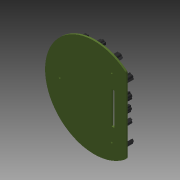
# Autodesk Inventor part: PCB
Saved by Autodesk Inventor 2015 (Build 190159000, 159)
## iProperties
Created: 2016-09-07
Part Number: PCB
Material: Generic
Document SubType Name: Modeling
Designer: James Yelland
Density: 1 g/cm^3
Appearance: Default
Author: James Yelland
Autodesk Inventor part; units mm, degrees
ref_plane "YZ Plane" through (0, 0, 0) normal (1, 0, 0) x (0, 1, 0)
ref_plane "XZ Plane" through (0, 0, 0) normal (0, 1, 0) x (-1, 0, 0)
ref_plane "XY Plane" through (0, 0, 0) normal (0, 0, 1) x (1, 0, 0)
sketch "Sketch4" plane through (0, 0, 0) normal (0, 1, 0) x (-1, 0, 0)
  line L0 (-55, 0) -> (-55, 62.45)
  line L1 (-55, 0) -> (-55, -62.45)
  arc A0 (-53.125, -66.3531) -> (-53.125, 66.3531) centre (0, 0) ccw
  arc A1 (-53.125, 66.3531) -> (-55, 62.45) centre (-50, 62.45) ccw
  arc A2 (-55, -62.45) -> (-53.125, -66.3531) centre (-50, -62.45) ccw
  circle A3 centre (-30.0153, 51.9527) radius 1.6
  circle A4 centre (60, 0) radius 1.6
  circle A5 centre (-30.0153, -51.9527) radius 1.6
  point P0 (-55, -64.8074)
  dimension "d56" = 3.2
  dimension "d57" = 3.2
  dimension "d58" = 3.2
  constraints: 7 point on circle, 6 centre point, 4 end point, 2 point on line
  measures "d56" diameter of A3
  measures "d57" diameter of A4
  measures "d58" diameter of A5
extrude "Extrusion2" add sketch "Sketch4" along normal blind 3
sketch "Sketch5" plane through (0, 3, 0) normal (0, 1, 0) x (1, 0, 0)
  line L0 (-78, 5) -> (-74, 5)
  line L1 (-74, 5) -> (-74, -5)
  line L2 (-74, -5) -> (-78, -5)
  arc A0 (-78, 2.5807) -> (-78, -2.5807) centre (-77.05, 0) ccw
  line L3 (-78, -5) -> (-78, -2.5807)
  line L4 (-78, 2.5807) -> (-78, 5)
  line L5 (-77.05, 0) -> (-85, 0)
  line L6 (-73.976, -25.2299) -> (-70.2805, -23.6992)
  line L7 (-70.2805, -23.6992) -> (-66.4537, -32.938)
  line L8 (-73.0502, -27.4651) -> (-73.976, -25.2299)
  line L9 (-66.4537, -32.938) -> (-70.1492, -34.4687)
  arc A1 (-73.0502, -27.4651) -> (-71.075, -32.2336) centre (-71.1849, -29.4858) ccw
  line L10 (-71.1849, -29.4858) -> (-78.5298, -32.5281)
  line L11 (-70.1492, -34.4687) -> (-71.075, -32.2336)
  line L12 (-58.6899, -51.6188) -> (-55.8614, -48.7904)
  line L13 (-55.8614, -48.7904) -> (-48.7904, -55.8614)
  line L14 (-56.9792, -53.3295) -> (-58.6899, -51.6188)
  line L15 (-48.7904, -55.8614) -> (-51.6188, -58.6899)
  arc A2 (-56.9792, -53.3295) -> (-53.3295, -56.9792) centre (-54.4826, -54.4826) ccw
  line L16 (-54.4826, -54.4826) -> (-60.1041, -60.1041)
  line L17 (-51.6188, -58.6899) -> (-53.3295, -56.9792)
  line L18 (-34.4687, -70.1492) -> (-32.938, -66.4537)
  line L19 (-32.938, -66.4537) -> (-23.6992, -70.2805)
  line L20 (-32.2336, -71.075) -> (-34.4687, -70.1492)
  line L21 (-23.6992, -70.2805) -> (-25.2299, -73.976)
  arc A3 (-32.2336, -71.075) -> (-27.4651, -73.0502) centre (-29.4858, -71.1849) ccw
  line L22 (-29.4858, -71.1849) -> (-32.5281, -78.5298)
  line L23 (-25.2299, -73.976) -> (-27.4651, -73.0502)
  line L24 (-5, -78) -> (-5, -74)
  line L25 (-5, -74) -> (5, -74)
  line L26 (-2.5807, -78) -> (-5, -78)
  line L27 (5, -74) -> (5, -78)
  arc A4 (-2.5807, -78) -> (2.5807, -78) centre (0, -77.05) ccw
  line L28 (0, -77.05) -> (0, -85)
  line L29 (5, -78) -> (2.5807, -78)
  line L30 (25.2299, -73.976) -> (23.6992, -70.2805)
  line L31 (23.6992, -70.2805) -> (32.938, -66.4537)
  line L32 (27.4651, -73.0502) -> (25.2299, -73.976)
  line L33 (32.938, -66.4537) -> (34.4687, -70.1492)
  arc A5 (27.4651, -73.0502) -> (32.2336, -71.075) centre (29.4858, -71.1849) ccw
  line L34 (29.4858, -71.1849) -> (32.5281, -78.5298)
  line L35 (34.4687, -70.1492) -> (32.2336, -71.075)
  line L36 (46.5147, -53.5858) -> (43.6863, -50.7574)
  line L37 (43.6863, -50.7574) -> (50.7574, -43.6863)
  line L38 (48.2254, -51.8751) -> (46.5147, -53.5858)
  line L39 (50.7574, -43.6863) -> (53.5858, -46.5147)
  arc A6 (48.2254, -51.8751) -> (51.8751, -48.2254) centre (49.3785, -49.3785) ccw
  line L40 (49.3785, -49.3785) -> (55, -55)
  line L41 (53.5858, -46.5147) -> (51.8751, -48.2254)
  line L42 (46.6194, -24.7224) -> (42.9239, -23.1916)
  line L43 (42.9239, -23.1916) -> (46.7507, -13.9528)
  line L44 (47.5453, -22.4872) -> (46.6194, -24.7224)
  line L45 (46.7507, -13.9528) -> (50.4463, -15.4836)
  arc A7 (47.5453, -22.4872) -> (49.5204, -17.7187) centre (47.6552, -19.7394) ccw
  line L46 (47.6552, -19.7394) -> (55, -22.7817)
  line L47 (50.4463, -15.4836) -> (49.5204, -17.7187)
  line L48 (48, -5) -> (44, -5)
  line L49 (44, -5) -> (44, 5)
  line L50 (48, -2.5807) -> (48, -5)
  line L51 (44, 5) -> (48, 5)
  arc A8 (48, -2.5807) -> (48, 2.5807) centre (47.05, 0) ccw
  line L52 (47.05, 0) -> (55, 0)
  line L53 (48, 5) -> (48, 2.5807)
  line L54 (50.4463, 15.4836) -> (46.7507, 13.9528)
  line L55 (46.7507, 13.9528) -> (42.9239, 23.1916)
  line L56 (49.5204, 17.7187) -> (50.4463, 15.4836)
  line L57 (42.9239, 23.1916) -> (46.6194, 24.7224)
  arc A9 (49.5204, 17.7187) -> (47.5453, 22.4872) centre (47.6552, 19.7394) ccw
  line L58 (47.6552, 19.7394) -> (55, 22.7817)
  line L59 (46.6194, 24.7224) -> (47.5453, 22.4872)
  line L60 (53.5858, 46.5147) -> (50.7574, 43.6863)
  line L61 (50.7574, 43.6863) -> (43.6863, 50.7574)
  line L62 (43.6863, 50.7574) -> (46.5147, 53.5858)
  arc A10 (51.8751, 48.2254) -> (48.2254, 51.8751) centre (49.3785, 49.3785) ccw
  line L63 (49.3785, 49.3785) -> (55, 55)
  line L64 (46.5147, 53.5858) -> (48.2254, 51.8751)
  line L65 (34.4687, 70.1492) -> (32.938, 66.4537)
  line L66 (32.938, 66.4537) -> (23.6992, 70.2805)
  line L67 (32.2336, 71.075) -> (34.4687, 70.1492)
  line L68 (23.6992, 70.2805) -> (25.2299, 73.976)
  arc A11 (32.2336, 71.075) -> (27.4651, 73.0502) centre (29.4858, 71.1849) ccw
  line L69 (29.4858, 71.1849) -> (32.5281, 78.5298)
  line L70 (25.2299, 73.976) -> (27.4651, 73.0502)
  line L71 (5, 78) -> (5, 74)
  line L72 (5, 74) -> (-5, 74)
  line L73 (2.5807, 78) -> (5, 78)
  line L74 (-5, 74) -> (-5, 78)
  arc A12 (2.5807, 78) -> (-2.5807, 78) centre (0, 77.05) ccw
  line L75 (0, 77.05) -> (0, 85)
  line L76 (-5, 78) -> (-2.5807, 78)
  line L77 (-25.2299, 73.976) -> (-23.6992, 70.2805)
  line L78 (-23.6992, 70.2805) -> (-32.938, 66.4537)
  line L79 (-27.4651, 73.0502) -> (-25.2299, 73.976)
  line L80 (-32.938, 66.4537) -> (-34.4687, 70.1492)
  arc A13 (-27.4651, 73.0502) -> (-32.2336, 71.075) centre (-29.4858, 71.1849) ccw
  line L81 (-29.4858, 71.1849) -> (-32.5281, 78.5298)
  line L82 (-34.4687, 70.1492) -> (-32.2336, 71.075)
  line L83 (-51.6188, 58.6899) -> (-48.7904, 55.8614)
  line L84 (-48.7904, 55.8614) -> (-55.8614, 48.7904)
  line L85 (-53.3295, 56.9792) -> (-51.6188, 58.6899)
  line L86 (-55.8614, 48.7904) -> (-58.6899, 51.6188)
  arc A14 (-53.3295, 56.9792) -> (-56.9792, 53.3295) centre (-54.4826, 54.4826) ccw
  line L87 (-54.4826, 54.4826) -> (-60.1041, 60.1041)
  line L88 (-58.6899, 51.6188) -> (-56.9792, 53.3295)
  line L89 (-70.1492, 34.4687) -> (-66.4537, 32.938)
  line L90 (-66.4537, 32.938) -> (-70.2805, 23.6992)
  line L91 (-71.075, 32.2336) -> (-70.1492, 34.4687)
  line L92 (-70.2805, 23.6992) -> (-73.976, 25.2299)
  arc A15 (-71.075, 32.2336) -> (-73.0502, 27.4651) centre (-71.1849, 29.4858) ccw
  line L93 (-71.1849, 29.4858) -> (-78.5298, 32.5281)
  line L94 (-73.976, 25.2299) -> (-73.0502, 27.4651)
  line L95 (55, -55) -> (49.8959, -49.8959)
  line L96 (55, 55) -> (49.8959, 49.8959)
  line L97 (53.5858, 46.5147) -> (51.8751, 48.2254)
  point P0 (0, 0)
  dimension "d52" = 4
  dimension "d53" = 10
  constraints: 196 end point, 32 point on circle, 16 centre point, 2 point on line, 1 perpendicular
  measures "d52" distance of L0.start L0.end
  measures "d53" distance of L0.end L1.end
extrude "Extrusion3" add sketch "Sketch5" along normal blind 12.5
sketch "Sketch6" plane through (0, 3, 0) normal (0, 1, 0) x (1, 0, 0)
  line L0 (55, -62.45) -> (55, 62.45) projected
  line L1 (55, 0) -> (35, 0)
  line L2 (35, 0) -> (35, -27)
  line L3 (35, 0) -> (35, 27)
  line L4 (34, 28) -> (31, 28)
  line L5 (30, 27) -> (30, -27)
  line L6 (31, -28) -> (34, -28)
  arc A0 (31, 28) -> (30, 27) centre (31, 27) ccw
  arc A1 (35, 27) -> (34, 28) centre (34, 27) ccw
  arc A2 (34, -28) -> (35, -27) centre (34, -27) ccw
  arc A3 (30, -27) -> (31, -28) centre (31, -27) ccw
  point P0 (0, 0)
  point P1 (35, -28)
  point P2 (35, 28)
  point P3 (30, 28)
  dimension "d59" = 20
  dimension "d60" = 28
  dimension "d61" = 28
  dimension "d62" = 5
  dimension "d63" = 1
  constraints: 12 end point, 8 point on circle, 8 tangent, 6 point on line, 4 centre point, 3 equal radius, 3 perpendicular, 2 horizontal, 1 midpoint, 1 vertical
  measures "d59" distance of L1.start L1.end
  measures "d60" distance of L1.end point (35, -28)
  measures "d61" distance of L1.end point (35, 28)
  measures "d62" distance of point (35, 28) point (30, 28)
  measures "d63" radius of A0
extrude "Extrusion4" cut sketch "Sketch6" against normal through all
body "Solid2"
